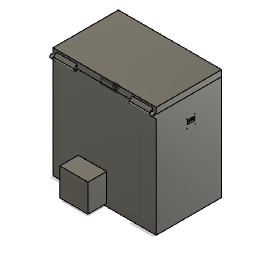
SmartTController v43 (Autodesk Fusion 360 design; units mm, degrees)
Autodesk Fusion 360 part; units mm, degrees
sketch "Sketch1" plane through (0, 0, 0) normal (0, 1, 0) x (1, 0, 0)
  line L0 (0, 0) -> (300, 0)
  line L1 (300, 0) -> (300, -190)
  line L2 (300, -190) -> (0, -190)
  line L3 (0, -190) -> (0, 0)
  line L4 (300, -50) -> (300, -115)
  dimension "d2" = 65
  constraint horizontal L0
  constraint vertical L1
  constraint horizontal L2
  constraint vertical L3
  constraint coincident L0.start L3.end
  constraint coincident L1 L4.start
  constraint parallel L1 L4
  measures "d2" distance of L4.start L4.end
extrude "Extrude1" add sketch "Sketch1" along normal blind 304 makes body 1
shell "Shell1" thickness 12 removed faces 1 at (100, 304, 101.6667) on bodies 1
sketch "Sketch2" plane through (0, 12, 0) normal (0, 1, 0) x (-1, 0, 0)
  line L0 (-288, 178) -> (-288, 12)
  line L1 (-288, 12) -> (-12, 12)
  line L2 (-12, 12) -> (-12, 178)
  line L3 (-12, 178) -> (-288, 178)
  circle A0 centre (-109.9013, 94.9089) radius 76.5
  dimension "d6" = 153
  measures "d6" diameter of A0
extrude "Extrude2" add sketch "Sketch2" along normal blind 7.6 contours A0 bodies 1
shell "Shell2" thickness 5 removed faces 1 at (135.1165, 19.6, 98.7095) on bodies 1
sketch "Sketch3" plane through (288, 0, 0) normal (-1, 0, 0) x (0, 0, 1)
  line L0 (12, 12) -> (178, 12)
  line L1 (178, 12) -> (178, 304)
  line L2 (178, 304) -> (12, 304)
  line L3 (12, 304) -> (12, 12)
  line L4 (12, 165) -> (178, 165)
  line L5 (95, 215.9288) -> (73, 215.9288)
  line L6 (73, 215.9288) -> (73, 226.9288)
  line L7 (73, 226.9288) -> (95, 226.9288)
  line L8 (95, 226.9288) -> (95, 215.9288)
  dimension "d10" = 22
  dimension "d11" = 11
  constraint coincident L3 L4.start
  constraint coincident L1 L4.end
  constraint perpendicular L1 L4
  constraint horizontal L5
  constraint vertical L6
  constraint horizontal L7
  constraint vertical L8
  measures "d10" distance of L5.start L5.end
  measures "d11" distance of L5.start L7.end
sketch "Sketch5" plane through (288, 0, 0) normal (-1, 0, 0) x (0, 0, 1)
  line L0 (12, 12) -> (178, 12)
  line L1 (178, 12) -> (178, 304)
  line L2 (178, 304) -> (12, 304)
  line L3 (12, 304) -> (12, 12)
  line L4 (75, 250) -> (102.3, 250)
  line L5 (102.3, 250) -> (102.3, 222.2)
  line L6 (102.3, 222.2) -> (75, 222.2)
  line L7 (75, 222.2) -> (75, 250)
  line L8 (75, 250) -> (75, 243.96)
  line L9 (75, 243.96) -> (77.73, 243.96)
  line L10 (77.73, 243.96) -> (99.47, 243.96)
  line L11 (99.47, 243.96) -> (99.47, 233.1)
  line L12 (99.47, 233.1) -> (77.73, 233.1)
  line L13 (77.73, 233.1) -> (77.73, 243.96)
  circle A0 centre (101, 248.5) radius 1.1
  circle A1 centre (76.2769, 248.7047) radius 1.1
  circle A2 centre (101, 223.7) radius 1.1
  circle A3 centre (76.2769, 223.4953) radius 1.1
  dimension "d14" = 27.3
  dimension "d15" = 27.8
  dimension "d16" = 6.04
  dimension "d17" = 2.73
  dimension "d18" = 21.74
  dimension "d19" = 10.86
  dimension "d20" = 2.2
  constraint horizontal L4
  constraint vertical L5
  constraint horizontal L6
  constraint vertical L7
  constraint perpendicular L4 L8
  constraint perpendicular L8 L9
  constraint horizontal L10
  constraint vertical L11
  constraint horizontal L12
  constraint vertical L13
  measures "d14" distance of L4.start L4.end
  measures "d15" distance of L4.start L6.end
  measures "d16" distance of L4.start L8.end
  measures "d17" distance of L8.end L9.end
  measures "d18" distance of L9.end L10.end
  measures "d19" distance of L9.end L12.end
  measures "d20" diameter of A0
extrude "Extrude4" cut sketch "Sketch5" against normal blind 70 contours L10 L11 L12 L13 | A0 | A1 | A2 | A3 bodies 1
sketch "Sketch6" plane through (0, 12, 0) normal (0, 1, 0) x (-1, 0, 0)
  circle A0 centre (-109.9013, 94.9089) radius 76.5
  line L0 (-288, 178) -> (-288, 12)
  line L1 (-288, 12) -> (-12, 12)
  line L2 (-12, 12) -> (-12, 178)
  line L3 (-12, 178) -> (-288, 178)
  line L4 (-288, 95) -> (-247, 95)
  line L5 (-233.5, 12) -> (-246.5, 12)
  line L6 (-246.5, 12) -> (-246.5, 178)
  line L7 (-246.5, 178) -> (-233.5, 178)
  line L8 (-233.5, 178) -> (-233.5, 12)
  line L9 (-233.5, 12) -> (-246.5, 178) construction
  line L10 (-246.5, 12) -> (-233.5, 178) construction
  point P0 (-240, 95)
  dimension "d23" = 41
  dimension "d24" = 13
  constraint midpoint L0 L4.start
  constraint perpendicular L0 L4
  constraint horizontal L5
  constraint perpendicular L5 L6
  constraint parallel L5 L7
  constraint parallel L6 L8
  constraint coincident L1 L5.start
  constraint coincident L9 P0
  constraint coincident L10 P0
  measures "d23" distance of L4.start L4.end
  measures "d24" distance of L6.end L7.end
extrude "Extrude5" add sketch "Sketch6" along normal blind 220 contours L1 L3 L5 L6 L7 L8 bodies 1
sketch "Sketch7" plane through (233.5, 0, 0) normal (-1, 0, 0) x (0, 0, 1)
  line L0 (12, 12) -> (178, 12)
  line L1 (178, 12) -> (178, 232)
  line L2 (178, 232) -> (12, 232)
  line L3 (12, 232) -> (12, 12)
  line L4 (51.4561, 12) -> (115.9721, 12)
  line L5 (115.9721, 12) -> (115.9721, 190.816)
  line L6 (115.9721, 190.816) -> (51.4561, 190.816)
  line L7 (51.4561, 190.816) -> (51.4561, 12)
  line L8 (51.4561, 12) -> (89.5561, 12)
  line L9 (89.5561, 12) -> (89.5561, 27.113)
  circle A0 centre (89.5561, 27.113) radius 3.55
  line L10 (89.5561, 27.113) -> (89.5561, 176.973)
  circle A1 centre (89.5561, 176.973) radius 3.55
  dimension "d28" = 64.516
  dimension "d29" = 178.816
  dimension "d30" = 38.1
  dimension "d31" = 15.113
  dimension "d32" = 7.1
  dimension "d33" = 149.86
  dimension "d34" = 7.1
  constraint horizontal L4
  constraint vertical L5
  constraint horizontal L6
  constraint vertical L7
  constraint coincident L0 L4.start
  constraint perpendicular L7 L8
  constraint perpendicular L8 L9
  constraint coincident L9.end A0.centre
  constraint parallel L9 L10
  constraint coincident L10.end A1.centre
  measures "d28" distance of L4.start L4.end
  measures "d29" distance of L4.start L6.end
  measures "d30" distance of L4.start L8.end
  measures "d31" distance of L8.end L9.end
  measures "d32" diameter of A0
  measures "d33" distance of L9.end L10.end
  measures "d34" diameter of A1
extrude "Extrude6" cut sketch "Sketch7" against normal blind 25 contours L9 A0 L10 | L9 A0 L10 | A1 bodies 1
sketch "Sketch8" plane through (233.5, 0, 0) normal (-1, 0, 0) x (0, 0, 1)
  circle A0 centre (89.5561, 176.973) radius 3.55
  circle A1 centre (89.5561, 27.113) radius 3.55
  line L0 (12, 12) -> (178, 12)
  line L1 (178, 12) -> (178, 232)
  line L2 (178, 232) -> (12, 232)
  line L3 (12, 232) -> (12, 12)
  line L4 (150, 160) -> (170, 160)
  line L5 (170, 160) -> (170, 60)
  line L6 (170, 60) -> (150, 60)
  line L7 (150, 60) -> (150, 160)
  constraint horizontal L4
  constraint vertical L5
  constraint horizontal L6
  constraint vertical L7
extrude "Extrude7" cut sketch "Sketch8" against normal blind 50 contours L4 L5 L6 L7 bodies 1
fillet "Fillet1" radius 6 2 edges at (246.5, 232, 95) (233.5, 232, 95) on bodies 1
sketch "Sketch9" plane through (0, 0, 12) normal (0, 0, 1) x (1, 0, 0)
  line L0 (12, 304) -> (12, 12)
  line L1 (12, 12) -> (233.5, 12)
  line L2 (233.5, 12) -> (233.5, 226)
  arc A0 (239.5, 232) -> (233.5, 226) centre (239.5, 226) ccw
  line L3 (239.5, 232) -> (240.5, 232)
  arc A1 (246.5, 226) -> (240.5, 232) centre (240.5, 226) ccw
  line L4 (246.5, 226) -> (246.5, 12)
  line L5 (246.5, 12) -> (288, 12)
  line L6 (288, 12) -> (288, 304)
  circle A2 centre (270, 80) radius 8
  line L7 (288, 304) -> (12, 304)
  dimension "d43" = 16
  measures "d43" diameter of A2
extrude "Extrude8" cut sketch "Sketch9" against normal blind 60 contours A2 bodies 1
sketch "Sketch17" plane through (0, 0, 190) normal (0, 0, 1) x (1, 0, 0)
  line L0 (0, 304) -> (0, 0)
  line L1 (0, 0) -> (300, 0)
  line L2 (300, 0) -> (300, 304)
  line L3 (0, 0) -> (230, 0)
  line L4 (115, 0) -> (115, 10)
  line L5 (115, 10) -> (76.9, 10)
  line L6 (115, 10) -> (153.1, 10)
  line L7 (76.9, 10) -> (153.1, 10)
  line L8 (153.1, 10) -> (153.1, 86.2)
  line L9 (153.1, 86.2) -> (76.9, 86.2)
  line L10 (76.9, 86.2) -> (76.9, 10)
  line L11 (300, 304) -> (0, 304)
  dimension "d62" = 10
  dimension "d63" = 38.1
  dimension "d64" = 76.2
  constraint coincident L0.end L1.start
  constraint coincident L1 L3.end
  constraint perpendicular L0 L3
  constraint vertical L4
  constraint midpoint L3 L4.start
  constraint perpendicular L4 L5
  constraint symmetric L5.start L4 L6.start
  constraint symmetric L4 L5.end L6.end
  constraint horizontal L7
  constraint vertical L8
  constraint horizontal L9
  constraint vertical L10
  measures "d62" distance of L4.start L4.end
  measures "d63" distance of L4.end L5.end
  measures "d64" distance of L5.end L9.end
extrude "Extrude15" cut sketch "Sketch17" against normal blind 40 contours L5 L6 L7 L8 L9 L10 bodies 1
sketch "Sketch18" plane through (0, 0, 190) normal (0, 0, 1) x (1, 0, 0)
  line L0 (73.9197, 88.4439) -> (155.8798, 88.4439)
  line L1 (155.8798, 88.4439) -> (155.8798, 7.7181)
  line L2 (155.8798, 7.7181) -> (73.9197, 7.7181)
  line L3 (73.9197, 7.7181) -> (73.9197, 88.4439)
  constraint horizontal L0
  constraint vertical L1
  constraint horizontal L2
  constraint vertical L3
extrude "Extrude16" add sketch "Sketch18" along normal blind 54 bodies 1
shell "Shell4" thickness 7 removed faces 1 at (127.7, 35.4, 190) on bodies 1
ref_plane "WorkPlane4" through (0, 304, 0) normal (0, -1, 0) x (1, 0, 0)
sketch "Sketch29" plane through (0, 304, 0) normal (0, -1, 0) x (1, 0, 0)
  line L0 (0, 0) -> (300, 0)
  line L1 (300, 0) -> (300, 190)
  line L2 (300, 190) -> (0, 190)
  line L3 (0, 190) -> (0, 0)
  constraint horizontal L0
  constraint vertical L1
  constraint horizontal L2
  constraint vertical L3
  constraint coincident L0.start L3.end
extrude "Extrude25" add sketch "Sketch29" against normal blind 17.78 bodies 1
split "Split2" by plane through (0, 304, 0) normal (0, -1, 0) bodies 1 makes body 2 at (87.5974, 129.157, 0)
sketch "Sketch30" plane through (300, 0, 0) normal (1, 0, 0) x (0, 0, -1)
  line L0 (0, 304) -> (-190, 304)
  line L1 (-190, 304) -> (-190, 0)
  line L2 (-190, 0) -> (0, 0)
  line L3 (0, 0) -> (0, 304)
  circle A0 centre (-101, 248.5) radius 1.1
  line L4 (-99.47, 233.1) -> (-99.47, 243.96)
  line L5 (-99.47, 243.96) -> (-77.73, 243.96)
  line L6 (-77.73, 243.96) -> (-77.73, 233.1)
  line L7 (-77.73, 233.1) -> (-99.47, 233.1)
  circle A1 centre (-101, 223.7) radius 1.1
  circle A2 centre (-76.2769, 248.7047) radius 1.1
  circle A3 centre (-76.2769, 223.4953) radius 1.1
  line L8 (-190, 304) -> (-190, 286.22) construction
  line L9 (-190, 304) -> (-225, 304) construction
  circle A4 centre (-195, 304) radius 1.5
  circle A5 centre (-195, 304) radius 1.7
  circle A6 centre (-195, 304) radius 4.7
  line L10 (-190, 304) -> (-190, 321.78)
  line L11 (-190, 304) -> (-190.3, 304)
  line L12 (-190, 315.6468) -> (-198.3234, 307.3234)
  line L13 (-190, 292.3532) -> (-198.3234, 300.6766)
  dimension "d101" = 17.78
  dimension "d102" = 3
  dimension "d103" = 0.2
  dimension "d104" = 3
  dimension "d105" = 5
  dimension "d106" = 45
  dimension "d107" = 45
  constraint coincident L0.end L1.start
  constraint perpendicular L0 L8
  constraint perpendicular L1 L9
  constraint coincident L9 A4.centre
  constraint concentric A4 A5
  constraint concentric A5 A6
  constraint coincident A6 L11.end
  constraint coincident L9 L11.end
  constraint coincident L10 L12.start
  constraint coincident A6 L12.end
  constraint tangent A6 L12
  constraint coincident L1 L13.start
  constraint coincident A6 L13.end
  constraint tangent A6 L13
  measures "d101" distance of L0.end L8.end
  measures "d102" diameter of A4
  measures "d103" distance of A4 A5
  measures "d104" distance of A5 A6
  measures "d105" distance of A4.centre L10
  measures "d106" angle of L10 L12
  measures "d107" angle of L8 L13
extrude "Extrude27" add sketch "Sketch30" against normal blind 9.5 contours L1 A6 L11 L13 | A6 | A4 | A5 bodies 2
extrude "Extrude28" add sketch "Sketch30" along normal blind 9.5 from surface at -300 contours L1 A6 L11 L13 | A6 | A4 | A5 bodies 2
extrude "Extrude29" cut sketch "Sketch30" against normal up to surface (300 mm away) contours A4 bodies 2
extrude "Extrude30" add sketch "Sketch30" against normal blind 60 from surface at -10 contours A6 L10 L11 L12 | A6 bodies 1
extrude "Extrude31" add sketch "Sketch30" along normal blind 60 from surface at -290 contours A6 L10 L11 L12 | A6 bodies 1
sketch "Sketch31" plane through (0, 0, 178) normal (0, 0, -1) x (-1, 0, 0)
  line L0 (-153.1, 12) -> (-153.1, 86.2)
  line L1 (-153.1, 86.2) -> (-76.9, 86.2)
  line L2 (-76.9, 86.2) -> (-76.9, 12)
  line L3 (-76.9, 12) -> (-12, 12)
  line L4 (-12, 12) -> (-12, 304)
  line L5 (-12, 304) -> (-288, 304)
  line L6 (-288, 304) -> (-288, 12)
  line L7 (-288, 12) -> (-246.5, 12)
  line L8 (-246.5, 12) -> (-246.5, 226)
  arc A0 (-240.5, 232) -> (-246.5, 226) centre (-240.5, 226) ccw
  line L9 (-240.5, 232) -> (-239.5, 232)
  arc A1 (-233.5, 226) -> (-239.5, 232) centre (-239.5, 226) ccw
  line L10 (-233.5, 226) -> (-233.5, 12)
  line L11 (-233.5, 12) -> (-153.1, 12)
  line L12 (-171, 304) -> (-129, 304)
  line L13 (-129, 304) -> (-129, 290)
  line L14 (-129, 290) -> (-171, 290)
  line L15 (-171, 290) -> (-171, 304)
  dimension "d123" = 42
  dimension "d124" = 14
  constraint horizontal L12
  constraint vertical L13
  constraint horizontal L14
  constraint vertical L15
  constraint coincident L5 L12.start
  constraint midpoint L5 L12
  measures "d123" distance of L12.start L12.end
  measures "d124" distance of L12.start L14.end
extrude "Extrude32" cut sketch "Sketch31" against normal blind 5 draft -45 contours L5 L12 L13 L14 L15 bodies 2
chamfer "Chamfer1" distance 2 angle 45 1 edges at (150, 304, 178) on bodies 2
extrude "Extrude35" add sketch "Sketch31" along normal blind 4 separate body contours L5 L12 L13 L14 L15 makes body 3
draft "Draft2" angle 60 neutral plane through (0, 0, 174) pull (0, 0, -1) 1 faces at (143, 304, 176.6667) on bodies 3
combine "Combine1" operation add target body 3 tool bodies 1
extrude "Extrude36" cut sketch "Sketch31" along normal blind 0.8 contours L5 L12 L13 L14 L15 bodies 3
extrude "Extrude37" add sketch "Sketch31" against normal blind 5 draft -45 from surface at 0.8 contours L5 L12 L13 L14 L15 bodies 3
fillet "Fillet3" radius 4 2 edges at (150, 299, 182.2) (150, 295, 182.2) on bodies 3
copy_body "Body->Comp1" bodies 3 removing the originals makes body 4 in component "Component"
copy_body "Body->Comp2" bodies 2 removing the originals makes body 5 in component "Box"
component "Component" placed x (1, 0, 0) y (0, 1, 0) z (0, 0, 1) at (0, 0, 0)
component "Box" placed x (1, 0, 0) y (0, 1, 0) z (0, 0, 1) at (0, 0, 0)
named bodies: "Lid", "Box"
